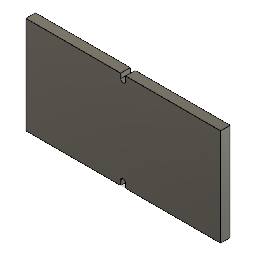
Table_17p1_Problem_1 (Autodesk Fusion 360 design; units mm, degrees)
Autodesk Fusion 360 part; units mm, degrees
sketch "Base_Surface" plane through (0, 0, 0) normal (0, 0, 1) x (1, 0, 0)
  line L0 (-100, 0) -> (-100, 50)
  line L1 (-100, 50) -> (-2.5, 50)
  line L2 (-2.5, 50) -> (-2.5, 45)
  arc A0 (-2.5, 45) -> (2.5, 45) centre (0, 45) ccw
  line L3 (2.5, 45) -> (2.5, 50)
  line L4 (2.5, 50) -> (100, 50)
  line L5 (100, 50) -> (100, 0)
  line L6 (-100, 0) -> (100, 0) construction
  line L7 (-100, 42.5) -> (100, 42.5) construction
  line L8 (0, 0) -> (0, 45) construction
  line L9 (-100, 0) -> (-100, -50)
  line L10 (-100, -50) -> (-2.5, -50)
  line L11 (2.5, -50) -> (100, -50)
  line L12 (100, -50) -> (100, 0)
  line L13 (2.5, -45) -> (2.5, -50)
  arc A1 (2.5, -45) -> (-2.5, -45) centre (0, -45) ccw
  line L14 (-2.5, -50) -> (-2.5, -45)
  dimension "Total_Width" = 200
  dimension "Notch_Radius" = 2.5
  dimension "Notch_Height" = 7.5
  dimension "Total_Height" = 100
  constraint vertical L0
  constraint perpendicular L0 L1
  constraint perpendicular L1 L2
  constraint tangent L2 A0
  constraint tangent A0 L3
  constraint parallel L0 L3
  constraint perpendicular L3 L4
  constraint perpendicular L4 L5
  constraint perpendicular L5 L6
  constraint equal L1 L4
  constraint coincident L0 L7.start
  constraint coincident L5 L7.end
  constraint perpendicular L5 L7
  constraint tangent A0 L7
  constraint equal L0 L5
  constraint coincident L8.start L6
  constraint coincident L8.start origin
  constraint coincident A0.centre L8.end
  constraint vertical L8
  constraint symmetric L0.start L6 L9.start
  constraint symmetric L0.end L6 L9.end
  constraint symmetric L1.end L6 L10.end
  constraint symmetric L2.end L6 A1.end
  constraint symmetric A0.end L6 L13.start
  constraint symmetric A0 L6 A1
  constraint symmetric L3.end L6 L11.start
  constraint symmetric L4.end L6 L11.end
  constraint symmetric L5.end L6 L12.end
  measures "Total_Width" distance of L0.start L5.end
  measures "Notch_Radius" radius of A0
  measures "Notch_Height" distance of L1 L7
  measures "Total_Height" distance of L1 L10
extrude "Extrude1" add sketch "Base_Surface" along normal mid plane 10
equation "Thickness = 1 cm"
